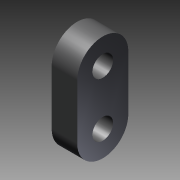
# Autodesk Inventor part: 205-S-ZS
Saved by Autodesk Inventor 2011 SP1 (Build 150282100, 282)
## iProperties
Created: 2017-03-01
Part Number: 205-S-ZS
Catalog Web Link: www.cadenas.de
Description: ZS-SU-Zwischenstuck
Vendor: DESTACO
Document SubType Name: Modeling
Designer: psAdmin
Manufacturer: DESTACO
Mass: 0.1722 g
Surface Area: 2.55551 cm^2
Volume: 0.1722 cm^3
Density: 1 g/cm^3
Category: PARTsolutions
Company: DESTACO
Title: 205-S-ZS
Author: Cadenas PARTsolutions
Comments: Zwischenstuck
PSOL_IDENT_0: {$CADENAS_DATA\23d-libs\destaco\destaco_gmbh\man_spann\horizontalspanner\standard\su_parts\zwischens
PSOL_IDENT_1: tuck_su.prj},150 {VTYP=3D},{NB=205-S-ZS},{LINA=205-S-ZS},{NN=ZS-SU},{DATE=20.09.2016 07:53:12},{GEOM
PSOL_IDENT_2: DATE=31.07.2006},{VERSION=v1},{LINEID=20},{LINESUBID=-1},{WBVAR=}  {NB=205-S-ZS},{LINA=205-S-ZS},{KT=
PSOL_IDENT_3: DUMMY},{MODELL=205-S-ZS},{SIZE=1},{MOD=1.000}
NN: ZS-SU
NT: Zwischenstuck
NB: 205-S-ZS
NBSYN: $MODELL.
LINA: 205-S-ZS
MODELL: 205-S-ZS
SIZE: 1
MOD: 1.000
SUPPLIER: DESTACO
ARTICLENO: 205-S-ZS
BOMINFO: 205-S-ZS
CREATOR: CADENAS GmbH
Autodesk Inventor part; units mm, degrees
sketch "Skizze_1" plane through (0, 0, 0) normal (1, 0, 0) x (0, 1, 0)
  arc A0 (3, 6.4) -> (-3, 6.4) centre (0, 6.4) ccw
  line L0 (-3, 6.4) -> (-3, 0)
  arc A1 (-3, 0) -> (3, 0) centre (0, 0) ccw
  line L1 (3, 0) -> (3, 6.4)
  constraints: 4 end point, 4 point on circle, 2 centre point
extrude "Extrusion1" add sketch "Skizze_1" along normal mid plane 3
sketch "Skizze_2" plane through (0, 0, 0) normal (0, 1, 0) x (-1, 0, 0)
  line L0 (-10, 0) -> (10, 0)
  line L1 (10, 0) -> (10, -1.215)
  line L2 (10, -1.215) -> (-10, -1.215)
  line L3 (-10, -1.215) -> (-10, 0)
  line L4 (-10, 0) -> (10, 0)
  constraints: 10 end point
revolve "Revolution1" cut sketch "Skizze_2" angle 360 about axis through (10, 0, 0) along (1, 0, 0)
sketch "Skizze_3" plane through (0, 0, 0) normal (0, 1, 0) x (-1, 0, 0)
  line L0 (-10, 6.4) -> (10, 6.4)
  line L1 (10, 6.4) -> (10, 5.185)
  line L2 (10, 5.185) -> (-10, 5.185)
  line L3 (-10, 5.185) -> (-10, 6.4)
  line L4 (-10, 6.4) -> (10, 6.4)
  constraints: 10 end point
revolve "Revolution2" cut sketch "Skizze_3" angle 360 about axis through (10, 0, 6.4) along (1, 0, 0)
ref_plane "ZS1_XY" through (0, 0, 0) normal (1, 0, 0) x (0, 0, -1)
ref_plane "ZS1_YZ" through (0, 0, 0) normal (0, 0, -1) x (0, 1, 0)
ref_plane "ZS1_ZX" through (0, 0, 0) normal (0, 1, 0) x (1, 0, 0)
ref_plane "ZS2_XY" through (0, 0, 6.4) normal (1, 0, 0) x (0, 0, -1)
ref_plane "ZS2_YZ" through (0, 0, 6.4) normal (0, 0, -1) x (0, 1, 0)
ref_plane "ZS2_ZX" through (0, 0, 6.4) normal (0, 1, 0) x (1, 0, 0)
body "Solid1"
